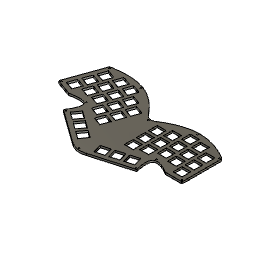
mrkabuda_switch_plate_unibody_19 v5 (Autodesk Fusion 360 design; units mm, degrees)
Autodesk Fusion 360 part; units mm, degrees
sketch "Sketch1" plane through (0, 0, 0) normal (0, 0, 1) x (1, 0, 0)
  line L0 (-56.8305, -43.5946) -> (3.7699, -26.1721)
  line L1 (32.056, -7.0618) -> (56.5101, -7.0618)
  line L2 (57.5101, -6.0618) -> (57.5101, 55.7146)
  line L3 (-39.2399, 50.5) -> (-25.2399, 50.5)
  line L4 (-25.2399, 50.5) -> (-25.2399, 36.5)
  line L5 (-25.2399, 36.5) -> (-39.2399, 36.5)
  line L6 (-39.2399, 36.5) -> (-39.2399, 50.5)
  line L7 (-39.2399, 31.5) -> (-25.2399, 31.5)
  line L8 (-25.2399, 31.5) -> (-25.2399, 17.5)
  line L9 (-25.2399, 17.5) -> (-39.2399, 17.5)
  line L10 (-39.2399, 17.5) -> (-39.2399, 31.5)
  line L11 (-39.2399, 12.5) -> (-25.2399, 12.5)
  line L12 (-25.2399, 12.5) -> (-25.2399, -1.5)
  line L13 (-25.2399, -1.5) -> (-39.2399, -1.5)
  line L14 (-39.2399, -1.5) -> (-39.2399, 12.5)
  line L15 (-6.2399, 17.7863) -> (-6.2399, 3.7863)
  line L16 (-20.2399, 17.7863) -> (-6.2399, 17.7863)
  line L17 (-6.2399, 3.7863) -> (-20.2399, 3.7863)
  line L18 (-6.2399, 36.7863) -> (-6.2399, 22.7863)
  line L19 (-6.2399, 22.7863) -> (-20.2399, 22.7863)
  line L20 (-6.2399, 55.7863) -> (-6.2399, 41.7863)
  line L21 (-20.2399, 41.7863) -> (-20.2399, 55.7863)
  line L22 (-20.2399, 22.7863) -> (-20.2399, 36.7863)
  line L23 (-20.2399, 36.7863) -> (-6.2399, 36.7863)
  line L24 (-6.2399, 41.7863) -> (-20.2399, 41.7863)
  line L25 (-20.2399, 55.7863) -> (-6.2399, 55.7863)
  line L26 (-20.2399, 3.7863) -> (-20.2399, 17.7863)
  line L27 (12.7601, 26.8291) -> (12.7601, 12.8291)
  line L28 (-1.2399, 26.8291) -> (12.7601, 26.8291)
  line L29 (12.7601, 12.8291) -> (-1.2399, 12.8291)
  line L30 (12.7601, 45.8291) -> (12.7601, 31.8291)
  line L31 (12.7601, 31.8291) -> (-1.2399, 31.8291)
  line L32 (12.7601, 64.8291) -> (12.7601, 50.8291)
  line L33 (-1.2399, 50.8291) -> (-1.2399, 64.8291)
  line L34 (-1.2399, 31.8291) -> (-1.2399, 45.8291)
  line L35 (-1.2399, 45.8291) -> (12.7601, 45.8291)
  line L36 (12.7601, 50.8291) -> (-1.2399, 50.8291)
  line L37 (-1.2399, 64.8291) -> (12.7601, 64.8291)
  line L38 (-1.2399, 12.8291) -> (-1.2399, 26.8291)
  line L39 (31.7601, 23.77) -> (31.7601, 9.77)
  line L40 (17.7601, 23.77) -> (31.7601, 23.77)
  line L41 (31.7601, 9.77) -> (17.7601, 9.77)
  line L42 (31.7601, 42.77) -> (31.7601, 28.77)
  line L43 (31.7601, 28.77) -> (17.7601, 28.77)
  line L44 (31.7601, 61.77) -> (31.7601, 47.77)
  line L45 (17.7601, 47.77) -> (17.7601, 61.77)
  line L46 (17.7601, 28.77) -> (17.7601, 42.77)
  line L47 (17.7601, 42.77) -> (31.7601, 42.77)
  line L48 (31.7601, 47.77) -> (17.7601, 47.77)
  line L49 (17.7601, 61.77) -> (31.7601, 61.77)
  line L50 (17.7601, 9.77) -> (17.7601, 23.77)
  line L51 (50.7601, 13.6882) -> (50.7601, -0.3118)
  line L52 (36.7601, 13.6882) -> (50.7601, 13.6882)
  line L53 (50.7601, -0.3118) -> (36.7601, -0.3118)
  line L54 (50.7601, 32.6882) -> (50.7601, 18.6882)
  line L55 (50.7601, 18.6882) -> (36.7601, 18.6882)
  line L56 (50.7601, 51.6882) -> (50.7601, 37.6882)
  line L57 (36.7601, 37.6882) -> (36.7601, 51.6882)
  line L58 (36.7601, 18.6882) -> (36.7601, 32.6882)
  line L59 (36.7601, 32.6882) -> (50.7601, 32.6882)
  line L60 (50.7601, 37.6882) -> (36.7601, 37.6882)
  line L61 (36.7601, 51.6882) -> (50.7601, 51.6882)
  line L62 (36.7601, -0.3118) -> (36.7601, 13.6882)
  line L63 (-57.0377, -22.0637) -> (-53.1694, -35.5187)
  line L64 (-53.1694, -35.5187) -> (-39.7144, -31.6504)
  line L65 (-39.7144, -31.6504) -> (-43.5827, -18.1954)
  line L66 (-43.5827, -18.1954) -> (-57.0377, -22.0637)
  line L67 (-38.7774, -16.8139) -> (-34.9091, -30.2689)
  line L68 (-34.9091, -30.2689) -> (-21.4541, -26.4006)
  line L69 (-21.4541, -26.4006) -> (-25.3224, -12.9456)
  line L70 (-25.3224, -12.9456) -> (-38.7774, -16.8139)
  line L71 (-7.0621, -7.6958) -> (-20.517, -11.5641)
  line L72 (-3.1938, -21.1508) -> (-7.0621, -7.6958)
  line L73 (-20.517, -11.5641) -> (-16.6488, -25.019)
  line L74 (-16.6488, -25.019) -> (-3.1938, -21.1508)
  arc A0 (30.9232, -6.9303) -> (32.056, -7.0618) centre (32.0625, -2.0618) ccw
  arc A1 (56.5101, -7.0618) -> (57.5101, -6.0618) centre (56.5101, -6.0618) ccw
  spline S0 degree 5 poles (4.4658, -24.9769) (4.0861, -23.4005) (3.405, -20.3536) (2.618, -16.1015) (2.0468, -11.0788) (2.1888, -5.9515) (3.2681, -2.0775) (5.3643, 0.4418) (8.517, 1.5538) (12.6793, 1.3152) (17.7712, -0.1754) (22.5239, -2.2909) (26.4446, -4.3657) (29.214, -5.9628) (30.6376, -6.8147) knots 0 0 0 0 0 0 0.1 0.2 0.3 0.4 0.5 0.6 0.7 0.8 0.9 1 1 1 1 1 1
  spline S1 degree 5 poles (-45.5293, 55.2274) (-43.5112, 56.5205) (-39.4737, 58.9944) (-33.4136, 62.369) (-25.324, 66.1865) (-15.1857, 69.7539) (-5.0083, 72.0179) (5.2193, 72.8785) (15.5025, 72.2743) (25.8353, 70.2596) (36.2064, 66.946) (44.5238, 63.3465) (50.7687, 60.1507) (54.9344, 57.8038) (57.0178, 56.5761) knots 0 0 0 0 0 0 0.1 0.2 0.3 0.4 0.5 0.6 0.7 0.8 0.9 1 1 1 1 1 1
  arc A2 (57.5101, 55.7146) -> (57.0178, 56.5761) centre (56.5101, 55.7146) ccw
  arc A3 (3.7699, -26.1721) -> (4.4658, -24.9769) centre (3.4936, -25.2111) ccw
  arc A4 (30.6376, -6.8147) -> (30.9232, -6.9303) centre (31.1511, -5.9566) ccw
  line L75 (6.3992, -33.0044) -> (2.5325, -16.9495)
  circle A5 centre (4.9998, 70.0097) radius 1.05
  line L76 (-4.8791, 72.3551) -> (14.8791, 72.6649)
  circle A6 centre (55.0101, 54.8574) radius 1.05
  line L77 (46.894, 62.5413) -> (67.1415, 50.611)
  circle A7 centre (55.0101, -4.5618) radius 1.05
  circle A8 centre (6.2551, 3.6516) radius 1.05
  circle A9 centre (1.6991, -24.1662) radius 1.05
  line L78 (3.2764, -1.6283) -> (7.7236, 1.6283)
  line L79 (-68.3458, 55.2892) -> (-81.5278, 60.0044)
  line L80 (-90.8545, 48.7759) -> (-104.0366, 53.4912)
  line L81 (-170.2011, 37.7583) -> (-157.0191, 33.0431)
  line L82 (-95.5698, 35.5939) -> (-90.8545, 48.7759)
  line L83 (-79.4603, 24.2172) -> (-74.745, 37.3993)
  line L84 (-87.9271, 42.1145) -> (-92.6423, 28.9325)
  line L85 (-99.6267, -19.3021) -> (-110.9928, -11.1282)
  line L86 (-91.4528, -7.9361) -> (-99.6267, -19.3021)
  line L87 (-95.5674, -22.2214) -> (-87.3935, -10.8554)
  line L88 (-115.1511, 22.4192) -> (-101.969, 17.704)
  line L89 (-102.8188, 0.2379) -> (-91.4528, -7.9361)
  line L90 (-87.3935, -10.8554) -> (-76.0275, -19.0293)
  line L91 (-110.9928, -11.1282) -> (-102.8188, 0.2379)
  line L92 (-99.0416, 11.0425) -> (-85.8595, 6.3273)
  line L93 (-106.8781, 3.1571) -> (-115.0521, -8.2089)
  line L94 (-76.0275, -19.0293) -> (-84.2014, -30.3953)
  line L95 (-118.2441, 11.3311) -> (-106.8781, 3.1571)
  line L96 (-84.2014, -30.3953) -> (-95.5674, -22.2214)
  line L97 (-97.2538, 30.886) -> (-110.4358, 35.6012)
  line L98 (-84.4553, 66.6659) -> (-97.6373, 71.3811)
  line L99 (-81.5278, 60.0044) -> (-86.2431, 46.8224)
  line L100 (-89.1705, 53.4838) -> (-84.4553, 66.6659)
  line L101 (-97.6373, 71.3811) -> (-102.3526, 58.1991)
  line L102 (-108.7518, 40.3091) -> (-95.5698, 35.5939)
  line L103 (-105.6988, 63.6897) -> (-118.8809, 68.4049)
  arc A10 (-154.8631, 25.1031) -> (-153.7523, 24.8454) centre (-153.1852, 29.8131) ccw
  circle A11 centre (-132.0407, -1.2263) radius 1.05
  line L104 (-152.3038, 46.2251) -> (-165.4859, 50.9404)
  line L105 (-85.8595, 6.3273) -> (-81.1443, 19.5093)
  line L106 (-102.3526, 58.1991) -> (-89.1705, 53.4838)
  line L107 (-101.969, 17.704) -> (-97.2538, 30.886)
  line L108 (-110.4358, 35.6012) -> (-115.1511, 22.4192)
  line L109 (-94.3263, 24.2246) -> (-99.0416, 11.0425)
  line L110 (-92.6423, 28.9325) -> (-79.4603, 24.2172)
  line L111 (-73.061, 42.1071) -> (-68.3458, 55.2892)
  line L112 (-104.0366, 53.4912) -> (-108.7518, 40.3091)
  line L113 (-81.1443, 19.5093) -> (-94.3263, 24.2246)
  line L114 (-74.745, 37.3993) -> (-87.9271, 42.1145)
  line L115 (-86.2431, 46.8224) -> (-73.061, 42.1071)
  line L116 (-145.9046, 64.1151) -> (-159.0866, 68.8303)
  line L117 (-122.935, 71.9165) -> (-118.2198, 85.0985)
  line L118 (-117.1968, 73.1128) -> (-104.0148, 68.3976)
  line L119 (-104.0148, 68.3976) -> (-99.2995, 81.5796)
  line L120 (-112.4816, 86.2949) -> (-117.1968, 73.1128)
  line L121 (-118.8809, 68.4049) -> (-123.5961, 55.2229)
  line L122 (-136.1171, 76.6317) -> (-122.935, 71.9165)
  line L123 (-124.619, 67.2086) -> (-137.8011, 71.9238)
  line L124 (-142.5163, 58.7418) -> (-129.3343, 54.0265)
  line L125 (-131.0183, 49.3186) -> (-144.2004, 54.0339)
  line L126 (-110.414, 50.5076) -> (-105.6988, 63.6897)
  circle A12 centre (-103.4299, 88.5591) radius 1.05
  line L127 (-157.4026, 73.5382) -> (-144.2205, 68.8229)
  line L128 (-123.5961, 55.2229) -> (-110.414, 50.5076)
  line L129 (-152.6874, 86.7202) -> (-157.4026, 73.5382)
  line L130 (-118.2198, 85.0985) -> (-131.4018, 89.8137)
  arc A13 (-156.9331, 93.4302) -> (-157.6869, 92.7848) centre (-156.7453, 92.448) ccw
  line L131 (-139.5053, 82.005) -> (-152.6874, 86.7202)
  line L132 (-144.2205, 68.8229) -> (-139.5053, 82.005)
  line L133 (-129.3343, 54.0265) -> (-124.619, 67.2086)
  line L134 (-99.2995, 81.5796) -> (-112.4816, 86.2949)
  line L135 (-137.8011, 71.9238) -> (-142.5163, 58.7418)
  circle A14 centre (-155.6216, 91.1357) radius 1.05
  line L136 (-131.4018, 89.8137) -> (-136.1171, 76.6317)
  line L137 (-112.0981, 45.7998) -> (-125.2801, 50.515)
  circle A15 centre (-175.6342, 35.188) radius 1.05
  line L138 (-157.0191, 33.0431) -> (-152.3038, 46.2251)
  arc A16 (-134.9188, -1.0578) -> (-134.6661, -2.4176) centre (-134.0823, -1.6057) ccw
  line L139 (-148.9156, 40.8518) -> (-135.7335, 36.1366)
  circle A17 centre (-126.9614, 26.5008) radius 1.05
  spline S2 degree 5 poles (-134.9188, -1.0578) (-134.0304, 0.2987) (-132.3629, 2.9381) (-130.1897, 6.6768) (-127.9602, 11.2136) (-126.367, 16.0892) (-126.0785, 20.1004) (-127.2037, 23.1785) (-129.7976, 25.2873) (-133.7972, 26.4645) (-139.0936, 26.776) (-144.2811, 26.3848) (-148.6716, 25.7517) (-151.817, 25.1807) (-153.4444, 24.858) knots 0 0 0 0 0 0 0.1 0.2 0.3 0.4 0.5 0.6 0.7 0.8 0.9 1 1 1 1 1 1
  line L140 (23.5387, -2.5663) -> (37.7364, -11.0631)
  line L141 (-139.4429, -7.9651) -> (-130.3948, 5.8495)
  line L142 (-125.935, 20.5261) -> (-129.0255, 25.0902)
  line L143 (-145.3294, 26.4673) -> (-161.5594, 23.2488)
  arc A18 (-178.4934, 34.6177) -> (-177.8886, 33.3393) centre (-177.5518, 34.2809) ccw
  line L144 (-163.8019, 55.6482) -> (-150.6198, 50.933)
  arc A19 (-153.7523, 24.8454) -> (-153.4444, 24.858) centre (-153.6389, 25.8389) ccw
  line L145 (-165.4859, 50.9404) -> (-170.2011, 37.7583)
  line L146 (-129.9954, 37.333) -> (-116.8133, 32.6177)
  line L147 (-154.8631, 25.1031) -> (-177.8886, 33.3393)
  line L148 (-125.2801, 50.515) -> (-129.9954, 37.333)
  line L149 (-115.0521, -8.2089) -> (-126.4181, -0.035)
  line L150 (-159.0866, 68.8303) -> (-163.8019, 55.6482)
  line L151 (-83.4742, -39.2326) -> (-134.6661, -2.4176)
  line L152 (-135.7335, 36.1366) -> (-131.0183, 49.3186)
  line L153 (-144.2004, 54.0339) -> (-148.9156, 40.8518)
  line L154 (-116.8133, 32.6177) -> (-112.0981, 45.7998)
  spline S3 degree 5 poles (-60.8315, 57.6221) (-62.2919, 59.5136) (-65.2529, 63.1936) (-69.8159, 68.4049) (-76.1464, 74.7256) (-84.4982, 81.5098) (-93.3276, 87.0789) (-102.6727, 91.3351) (-112.5536, 94.2273) (-122.9479, 95.8117) (-133.8166, 96.1878) (-142.8601, 95.6016) (-149.8263, 94.6947) (-154.5508, 93.8858) (-156.9331, 93.4302) knots 0 0 0 0 0 0 0.1 0.2 0.3 0.4 0.5 0.6 0.7 0.8 0.9 1 1 1 1 1 1
  line L155 (-53.6938, 48.3769) -> (-67.9693, 66.8673)
  line L156 (-93.3382, 87.4402) -> (-111.8376, 94.3865)
  line L157 (-145.3918, 95.6372) -> (-168.4745, 91.2233)
  line L158 (-178.4934, 34.6177) -> (-157.6869, 92.7848)
  line L159 (-150.6198, 50.933) -> (-145.9046, 64.1151)
  line L160 (-126.4181, -0.035) -> (-118.2441, 11.3311)
  spline S4 degree 5 poles (-83.4742, -39.2326) (-82.9534, -39.586) (-81.9108, -40.2698) (-80.3437, -41.2265) (-78.2479, -42.3619) (-75.6167, -43.5314) (-72.9733, -44.4279) (-70.3163, -45.0278) (-67.6452, -45.3159) (-64.9604, -45.3013) (-62.2628, -45.0056) (-60.0954, -44.562) (-58.4648, -44.1201) (-57.3756, -43.7777) (-56.8305, -43.5946) knots 0 0 0 0 0 0 0.1 0.2 0.3 0.4 0.5 0.6 0.7 0.8 0.9 1 1 1 1 1 1
  spline S5 degree 5 poles (-60.8315, 57.6221) (-60.55, 57.3408) (-59.9847, 56.7985) (-59.1303, 56.0457) (-57.9783, 55.1657) (-56.5152, 54.2858) (-55.0269, 53.646) (-53.5113, 53.2666) (-51.9672, 53.1598) (-50.3955, 53.3162) (-48.7983, 53.7166) (-47.5016, 54.2163) (-46.5193, 54.6857) (-45.86, 55.04) (-45.5293, 55.2274) knots 0 0 0 0 0 0 0.1 0.2 0.3 0.4 0.5 0.6 0.7 0.8 0.9 1 1 1 1 1 1
  circle A20 centre (-70, -42.5) radius 1.05
  circle A21 centre (-53.6938, 50.8199) radius 1.05
  point P0 (5.5, 0)
  point P1 (5, 72.51)
  point P2 (-122.3016, 20.9558)
  point P3 (-127.4803, 22.8082)
  point P4 (-102.5879, 90.9134)
  point P5 (-70, -45)
  point P6 (-53.4083, 53.3199)
  dimension "d2" = 14
  dimension "d3" = 14
  dimension "d4" = 14
  dimension "d5" = 14
  dimension "d6" = 14
  dimension "d7" = 14
  dimension "d18" = 14
  dimension "d19" = 14
  dimension "d20" = 14
  dimension "d21" = 14
  dimension "d22" = 14
  dimension "d23" = 14
  dimension "d26" = 14
  dimension "d27" = 14
  dimension "d28" = 14
  dimension "d29" = 14
  dimension "d30" = 14
  dimension "d31" = 14
  dimension "d34" = 14
  dimension "d35" = 14
  dimension "d36" = 14
  dimension "d37" = 14
  dimension "d38" = 14
  dimension "d39" = 14
  dimension "d42" = 14
  dimension "d43" = 14
  dimension "d44" = 14
  dimension "d45" = 14
  dimension "d46" = 14
  dimension "d47" = 14
  dimension "d48" = 5
  dimension "d50" = 5
  dimension "d51" = 5
  dimension "d52" = 5
  dimension "d53" = 5
  dimension "d54" = 5
  dimension "d55" = 5
  dimension "d59" = 5
  dimension "d66" = 14
  dimension "d67" = 14
  dimension "d70" = 14
  dimension "d71" = 14
  dimension "d73" = 14
  dimension "d74" = 14
  dimension "d80" = 1
  dimension "d139" = 1
  dimension "d141" = 1
  dimension "d142" = 1
  dimension "d178" = 2.1
  dimension "d179" = 2.5
  dimension "d180" = 2.1
  dimension "d181" = 2.5
  dimension "d182" = 2.5
  dimension "d183" = 2.1
  dimension "d184" = 2.5
  dimension "d185" = 2.5
  dimension "d186" = 2.1
  dimension "d187" = 2.1
  dimension "d188" = 2.5
  dimension "d189" = 2.5
  dimension "d190" = 2.5
  dimension "d201" = 5
  dimension "d202" = 6.75
  dimension "d203" = 6.75
  dimension "d204" = 5
  dimension "d205" = 5
  dimension "d206" = 5
  dimension "d207" = 5
  dimension "d208" = 5
  dimension "d209" = 5
  dimension "d210" = 5
  dimension "d211" = 5
  dimension "d212" = 5
  dimension "d214" = 5
  dimension "d215" = 5
  dimension "d216" = 2.1
  dimension "d217" = 2.5
  dimension "d218" = 2.1
  dimension "d219" = 2.5
  constraint horizontal L1
  constraint perpendicular L1 L2
  constraint horizontal L3
  constraint vertical L4
  constraint horizontal L5
  constraint vertical L6
  constraint horizontal L7
  constraint vertical L8
  constraint horizontal L9
  constraint vertical L10
  constraint horizontal L11
  constraint vertical L12
  constraint horizontal L13
  constraint vertical L14
  constraint horizontal L25
  constraint vertical L20
  constraint horizontal L24
  constraint vertical L21
  constraint horizontal L23
  constraint vertical L18
  constraint horizontal L19
  constraint vertical L22
  constraint horizontal L16
  constraint vertical L15
  constraint horizontal L17
  constraint vertical L26
  constraint horizontal L37
  constraint vertical L32
  constraint horizontal L36
  constraint vertical L33
  constraint horizontal L35
  constraint vertical L30
  constraint horizontal L31
  constraint vertical L34
  constraint horizontal L28
  constraint vertical L27
  constraint horizontal L29
  constraint vertical L38
  constraint horizontal L49
  constraint vertical L44
  constraint horizontal L48
  constraint vertical L45
  constraint horizontal L47
  constraint vertical L42
  constraint horizontal L43
  constraint vertical L46
  constraint horizontal L40
  constraint vertical L39
  constraint horizontal L41
  constraint vertical L50
  constraint horizontal L61
  constraint vertical L56
  constraint horizontal L60
  constraint vertical L57
  constraint horizontal L59
  constraint vertical L54
  constraint horizontal L55
  constraint vertical L58
  constraint horizontal L52
  constraint vertical L51
  constraint horizontal L53
  constraint vertical L62
  constraint perpendicular L63 L64
  constraint parallel L63 L65
  constraint parallel L64 L66
  constraint perpendicular L67 L68
  constraint parallel L67 L69
  constraint parallel L68 L70
  constraint parallel L65 L67
  constraint parallel L0 L64
  constraint perpendicular L73 L74
  constraint parallel L72 L73
  constraint parallel L71 L74
  constraint collinear L70 L71
  constraint collinear L66 L70
  constraint tangent L2 A2
  constraint tangent S1 A2
  constraint tangent L0 A3
  constraint tangent S0 A3
  constraint tangent A0 A4
  constraint tangent S0 A4
  constraint midpoint S0.start L75
  constraint midpoint P1 L76
  constraint midpoint S1.end L77
  constraint midpoint P0 L78
  constraint collinear L54 L56
  constraint collinear L51 L54
  constraint collinear L42 L44
  constraint collinear L39 L42
  constraint midpoint S0.end L140
  measures "d2" distance of L3.start L3.end
  measures "d3" distance of L3.start L5.end
  measures "d4" distance of L7.start L9.end
  measures "d5" distance of L7.start L7.end
  measures "d6" distance of L11.start L11.end
  measures "d7" distance of L11.start L13.end
  measures "d18" distance of L21.end L20.start
  measures "d19" distance of L21.end L21.start
  measures "d20" distance of L22.end L19.end
  measures "d21" distance of L18.start L22.end
  measures "d22" distance of L15.start L16.start
  measures "d23" distance of L17.end L16.start
  measures "d26" distance of L33.end L32.start
  measures "d27" distance of L33.end L33.start
  measures "d28" distance of L34.end L31.end
  measures "d29" distance of L30.start L34.end
  measures "d30" distance of L27.start L28.start
  measures "d31" distance of L29.end L28.start
  measures "d34" distance of L45.end L44.start
  measures "d35" distance of L45.end L45.start
  measures "d36" distance of L46.end L43.end
  measures "d37" distance of L42.start L46.end
  measures "d38" distance of L39.start L40.start
  measures "d39" distance of L41.end L40.start
  measures "d42" distance of L57.end L56.start
  measures "d43" distance of L57.end L57.start
  measures "d44" distance of L58.end L55.end
  measures "d45" distance of L54.start L58.end
  measures "d46" distance of L51.start L52.start
  measures "d47" distance of L53.end L52.start
  measures "d48" distance of L59 L60
  measures "d50" distance of L4 L21
  measures "d51" distance of L8 L22
  measures "d52" distance of L12 L26
  measures "d53" distance of L20 L33
  measures "d54" distance of L18 L34
  measures "d55" distance of L15 L38
  measures "d59" distance of L44 L57
  measures "d66" distance of L63.start L63.end
  measures "d67" distance of L63.start L65.end
  measures "d70" distance of L67.start L67.end
  measures "d71" distance of L67.start L69.end
  measures "d73" distance of L71.end L73.end
  measures "d74" distance of L71.end L71.start
  measures "d80" radius of A1
  measures "d139" radius of A2
  measures "d141" radius of A3
  measures "d142" radius of A4
  measures "d178" diameter of A5
  measures "d179" distance of A5.centre L76
  measures "d180" diameter of A6
  measures "d181" distance of L2 A6.centre
  measures "d182" distance of A6.centre L77
  measures "d183" diameter of A7
  measures "d184" distance of L2 A7.centre
  measures "d185" distance of L1 A7.centre
  measures "d186" diameter of A8
  measures "d187" diameter of A9
  measures "d188" distance of A8.centre L78
  measures "d189" distance of L0 A9.centre
  measures "d190" distance of L75 A9.centre
  measures "d201" distance of L52 L55
  measures "d202" distance of L1 L53
  measures "d203" distance of L2 L56
  measures "d204" distance of L32 L45
  measures "d205" distance of L47 L48
  measures "d206" distance of L40 L43
  measures "d207" distance of L28 L31
  measures "d208" distance of L35 L36
  measures "d209" distance of L23 L24
  measures "d210" distance of L16 L19
  measures "d211" distance of L5 L7
  measures "d212" distance of L9 L11
  measures "d214" distance of L65 L67
  measures "d215" distance of L69 L73
  measures "d216" diameter of A20
  measures "d217" distance of P5 A20.centre
  measures "d218" diameter of A21
  measures "d219" vertical distance of P6 A21.centre
extrude "Extrude3" add sketch "Sketch1" along normal blind 3
